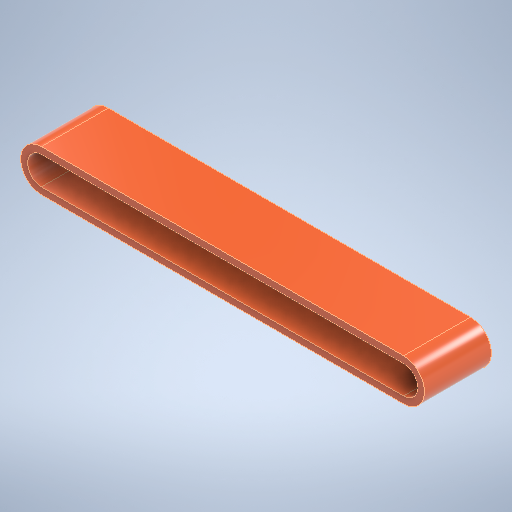
# Autodesk Inventor part: Conveyor_003_001
Saved by Autodesk Inventor 2026 (Build 300175000, 175)
## iProperties
Created: 2025-05-22
Part Number: Conveyor_003_001
Material: Rubber
Document SubType Name: Modeling
Designer: carlo
Density: 0.93 g/cm^3
Appearance: Smooth - Light Orange
Author: carlo
Autodesk Inventor part; units mm, degrees
ref_plane "YZ Plane" through (0, 0, 0) normal (1, 0, 0) x (0, 1, 0)
ref_plane "XZ Plane" through (0, 0, 0) normal (0, 1, 0) x (-1, 0, 0)
ref_plane "XY Plane" through (0, 0, 0) normal (0, 0, 1) x (1, 0, 0)
sketch "Sketch1" plane through (0, 0, 0) normal (0, 0, 1) x (1, 0, 0)
  line L0 (-130, 15) -> (130, 15)
  circle A0 centre (130, 0) radius 15 construction
  arc A1 (130, -15) -> (130, 15) centre (130, 0) ccw
  line L1 (-130, -15) -> (130, -15)
  arc A2 (-130, 15) -> (-130, -15) centre (-130, 0) ccw
  line L2 (130, 10) -> (-130, 10)
  arc A3 (-130, 10) -> (-130, -10) centre (-130, 0) ccw
  line L3 (-130, -10) -> (130, -10)
  arc A4 (130, -10) -> (130, 10) centre (130, 0) ccw
  point P0 (0, 0)
  point P1 (0, 15)
  dimension "d0" = 260
  dimension "d3" = 5
  dimension "d6" = 10
  dimension "d7" = 20
  constraints: 8 end point, 8 point on circle, 4 centre point, 3 horizontal, 2 tangent, 2 vertical alignment, 1 horizontal alignment, 1 midpoint, 1 parallel, 6 other
  measures "d0" distance of L0.start L0.end
  measures "d3" distance between parallel lines of L0 L2
  measures "d6" distance from line of point (0, 0) L2
  measures "d7" distance between parallel lines of L2 L3
extrude "Extrusion1" add sketch "Sketch1" along normal mid plane 48
body "Solid1"
